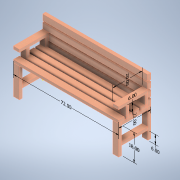
# Autodesk Inventor part: bench
Saved by Autodesk Inventor 2022 (Build 260153000, 153)
## iProperties
Created: 2023-03-06
Part Number: bench
Material: Wood (Oak)
Document SubType Name: Modeling
Designer: 0612003245
Density: 0.76 g/cm^3
Appearance: White Oak - Natural Medium Gloss
Author: 0612003245
Autodesk Inventor part; units mm, degrees
ref_plane "YZ Plane" through (0, 0, 0) normal (1, 0, 0) x (0, 1, 0)
ref_plane "XZ Plane" through (0, 0, 0) normal (0, 1, 0) x (-1, 0, 0)
ref_plane "XY Plane" through (0, 0, 0) normal (0, 0, 1) x (1, 0, 0)
sketch "Sketch1" plane through (0, 0, 0) normal (0, 0, 1) x (1, 0, 0)
  line L0 (0, 0) -> (0, 508)
  line L1 (0, 508) -> (101.6, 508)
  line L2 (101.6, 508) -> (101.6, 0)
  line L3 (101.6, 0) -> (0, 0)
  dimension "d0" = 508
  dimension "d1" = 101.6
  constraints: 8 end point, 3 perpendicular, 1 vertical
  measures "d0" distance of L0.start L0.end
  measures "d1" distance of L0.end L1.end
extrude "Extrusion1" add sketch "Sketch1" along normal blind 50.8
pattern_linear "Rectangular Pattern1" count 2 spacing 508 along (0, 0, 1) count 2 spacing 1727.2 along (1, 0, 0) of "Extrusion1"
sketch "Sketch2" plane through (0, 0, 50.8) normal (0, 0, 1) x (1, 0, 0)
  line L0 (0, 508) -> (0, 0) projected
  line L1 (0, 152.4) -> (101.6, 152.4)
  line L2 (101.6, 0) -> (101.6, 508) projected
  line L3 (0, 152.4) -> (0, 203.2)
  line L4 (0, 203.2) -> (101.6, 203.2)
  line L5 (101.6, 203.2) -> (101.6, 152.4)
  line L6 (0, 0) -> (101.6, 0) projected
  dimension "d10" = 50.8
  dimension "d11" = 152.4
  constraints: 8 end point, 3 perpendicular, 2 point on line, 1 horizontal
  measures "d10" distance of L1.start L3.end
  measures "d11" distance between parallel lines of L6 L1
extrude "Extrusion2" add sketch "Sketch2" along normal up to surface (457.2 mm away) separate body contours L4 L2 L1 L0
pattern_linear "Rectangular Pattern2" count 2 spacing 1727.2 along (1, 0, 0) count 2 spacing 304.8 along (0, 1, 0) of "Extrusion2" bodies 2
sketch "Sketch3" plane through (1727.2, 508, 50.8) normal (0, 0, 1) x (1, 0, 0)
  point P0 (-1727.2, -508)
sketch "Sketch4" plane through (0, 508, 508) normal (0, 1, 0) x (1, 0, 0)
  point P0 (0, 508)
sketch "Sketch5" plane through (0, 508, 508) normal (0, 1, 0) x (1, 0, 0)
  line L0 (0, 0) -> (0, -50.8) projected
  line L1 (0, -50.8) -> (1828.8, -50.8)
  line L2 (1828.8, -50.8) -> (1828.8, 50.8)
  line L3 (1828.8, 457.2) -> (1828.8, 0) projected
  line L4 (1828.8, 50.8) -> (0, 50.8)
  line L5 (0, 457.2) -> (0, 0) projected
  point P0 (0, 508)
  dimension "d20" = 101.6
  constraints: 6 end point, 2 point on line, 1 perpendicular
  measures "d20" distance of L1.end L2.end
extrude "Extrusion3" add sketch "Sketch5" along normal blind 50.8 separate body
pattern_linear "Rectangular Pattern3" count 4 spacing 127 along (0, 0, -1) of "Extrusion3" bodies 3
sketch "Sketch6" plane through (1727.2, 508, 0) normal (0, 1, 0) x (1, 0, 0)
  line L0 (-1727.2, 0) -> (-1727.2, -50.8) projected
  line L1 (-1727.2, -50.8) -> (-1625.6, -50.8) projected
  line L2 (-1727.2, -50.8) -> (-1625.6, -50.8)
  line L3 (-1625.6, -50.8) -> (-1625.6, -101.6)
  line L4 (-1625.6, -50.8) -> (-1625.6, -508) projected
  line L5 (-1625.6, -101.6) -> (-1727.2, -101.6)
  line L6 (-1727.2, -50.8) -> (-1727.2, -508) projected
  line L7 (-1727.2, -50.8) -> (-1727.2, -101.6)
  line L8 (-1727.2, -101.6) -> (-1625.6, -101.6)
  dimension "d26" = 50.8
  dimension "d27" = 50.8
  constraints: 10 end point, 2 perpendicular, 2 point on line, 1 collinear, 1 horizontal
  measures "d26" distance of L1.end L3.end
  measures "d27" distance of L0.end L5.end
extrude "Extrusion4" add sketch "Sketch6" along normal blind 203.2 separate body
pattern_linear "Rectangular Pattern4" count 2 spacing 330.2 along (0, 0, 1) count 2 spacing 1727.2 along (1, 0, 0) of "Extrusion4" bodies 4
sketch "Sketch10" plane through (1727.2, 711.2, 0) normal (0, 1, 0) x (1, 0, 0)
  line L0 (101.6, -50.8) -> (-1727.2, -50.8) projected
  line L1 (-1727.2, -508) -> (-1727.2, -558.8) projected
  line L2 (-1727.2, -50.8) -> (-1727.2, -558.8)
  line L3 (-1727.2, -558.8) -> (-1625.6, -558.8)
  line L4 (-1625.6, -101.6) -> (-1625.6, -50.8) projected
  line L5 (-1625.6, -558.8) -> (-1625.6, -50.8)
  point P0 (-1727.2, 0)
  constraints: 6 end point, 2 perpendicular, 1 collinear
extrude "Extrusion7" add sketch "Sketch10" along normal blind 50.8 separate body
pattern_linear "Rectangular Pattern7" count 2 spacing 1727.2 along (1, 0, 0) of "Extrusion7" bodies 5
sketch "Sketch11" plane through (1727.2, 508, 0) normal (0, 1, 0) x (1, 0, 0)
  line L0 (-1727.2, 0) -> (-1727.2, -50.8) projected
  line L1 (101.6, 0) -> (101.6, -50.8) projected
  line L2 (-1727.2, 0) -> (101.6, 0)
  line L3 (101.6, 0) -> (96.9046, -50.8)
  line L4 (-1727.2, 0) -> (-1727.2, -50.8) projected
  line L5 (96.9046, -50.8) -> (-1727.2, -50.8)
  constraints: 6 end point, 1 horizontal, 1 perpendicular
extrude "Extrusion8" add sketch "Sketch11" along normal blind 101.6 separate body
pattern_linear "Rectangular Pattern8" count 4 spacing 127 along (0, 1, 0) of "Extrusion8" bodies 6
body "Solid1"
body "Solid2"
body "Solid3"
body "Solid4"
body "Solid7"
body "Solid8"
